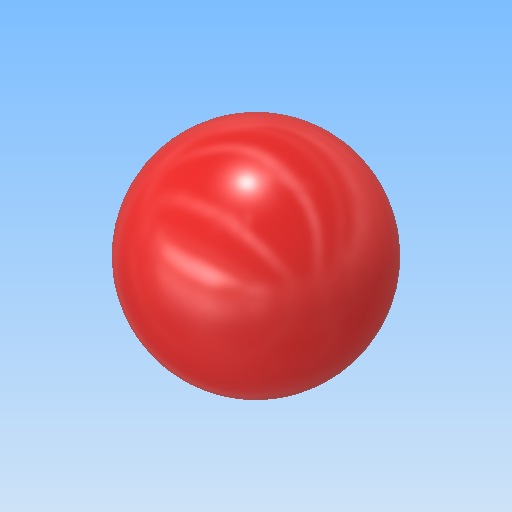
# Autodesk Inventor part: Ball 30mm
Saved by Autodesk Inventor 2018.1 (Build 221171000, 171)
## iProperties
Created: 2019-02-18
Part Number: Ball 30mm
Material: Copper, Alloy
Document SubType Name: Modeling
Designer: James
Density: 8.92 g/cm^3
Appearance: Light Red
Mass: 126.104 g
Surface Area: 28.2743 cm^2
Volume: 14.1372 cm^3
Author: James
Autodesk Inventor part; units mm, degrees
ref_plane "YZ Plane" through (0, 0, 0) normal (1, 0, 0) x (0, 1, 0)
ref_plane "XZ Plane" through (0, 0, 0) normal (0, 1, 0) x (-1, 0, 0)
ref_plane "XY Plane" through (0, 0, 0) normal (0, 0, 1) x (1, 0, 0)
sketch "Sketch1" plane through (0, 0, 0) normal (0, 0, 1) x (1, 0, 0)
  circle A0 centre (0, 0) radius 15
  dimension "d0" = 30
  constraints: 1 centre point, 1 coincident
  measures "d0" diameter of A0
extrude "Extrusion1" add sketch "Sketch1" along normal mid plane 30
fillet "Fillet1" radius 15 2 edges at (-15, 0, 15) (-15, 0, -15)
body "Solid1"
